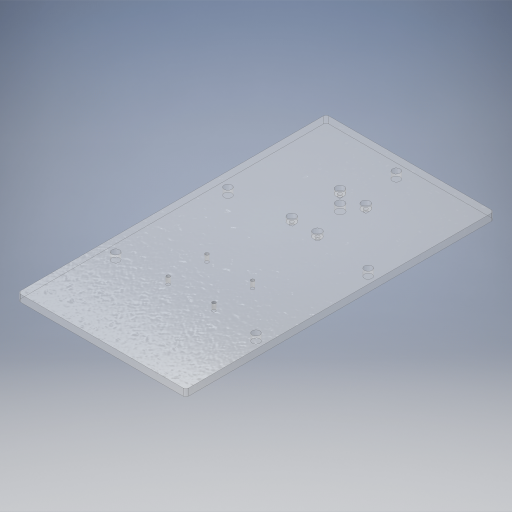
# Autodesk Inventor part: BT002_trajan20_21
Saved by Autodesk Inventor 2023 (Build 270158000, 158)
## iProperties
Company: HTBLA Kaindorf
RuleStatus: InUse
Created: 2022-08-03
Part Number: BT002_trajan20_21
Project: Zeichenmaschine_v2
Material: Acryl
Description: Platte Getriebemotor
Document SubType Name: Modeling
Designer: trajan20
Density: 1.188 g/cm^3
Appearance: Transparent - farblos
Mass: 155.33 g
Surface Area: 567.811 cm^2
Volume: 130.749 cm^3
AfterDocNew0: iProperties-Editor_aufrufen
Author: jan
Keywords: 2021
Autodesk Inventor part; units mm, degrees
ref_plane "YZ Plane" through (0, 0, 0) normal (1, 0, 0) x (0, 1, 0)
ref_plane "XZ Plane" through (0, 0, 0) normal (0, 1, 0) x (-1, 0, 0)
ref_plane "XY Plane" through (0, 0, 0) normal (0, 0, 1) x (1, 0, 0)
derived "BT000_trajan20_22_Zeichenmaschine_neu_Masterskizze.ipt"
sketch "Skizze3" plane through (0, 0, 0) normal (0, 0, 1) x (1, 0, 0)
  line L0 (0, 0) -> (-110, 0)
  line L1 (-220, 0) -> (-220, 120)
  line L2 (-220, 120) -> (0, 120)
  line L3 (0, 120) -> (0, 0)
  line L4 (-248.2253, 60) -> (-229.9902, 60) construction
  line L5 (-179.05, 50.815) -> (-179.05, 69.185) construction
  line L6 (-179.05, 69.185) -> (-144.68, 69.185) construction
  line L7 (-144.68, 50.3276) -> (-144.68, 69.185) construction
  line L8 (-143.2541, 50.815) -> (-179.05, 50.815) construction
  circle A0 centre (-170, 60) radius 3
  line L9 (-95, 40) -> (-70, 40)
  line L10 (-70, 40) -> (-70, 80)
  line L11 (-70, 80) -> (-95, 80)
  line L12 (-95, 80) -> (-95, 40)
  line L13 (-110, -37.5982) -> (-110, -22.8575) construction
  line L14 (-110, 0) -> (-220, 0)
  circle A1 centre (-170, 60) radius 20.5
  point P0 (-220, 60)
  point P1 (-144.68, 50.815)
  point P2 (-95, 60)
  point P3 (-91.3, 43.7)
  point P4 (-210, 60)
  point P5 (-110, 120)
  point P6 (-165, 0)
  point P7 (-60, 10)
  point P8 (-140, 10)
  point P9 (-140, 110)
  point P10 (-60, 110)
  point P11 (-60, 10)
  dimension "d4" = 120
  dimension "d5" = 220
  dimension "d6" = 50
  dimension "d8" = 9.05
  dimension "d9" = 34.37
  dimension "d11" = 9.185
  dimension "d12" = 18.37
  dimension "d17" = 6
  dimension "d18" = 40
  dimension "d19" = 25
  dimension "d20" = 75
  dimension "d21" = 3.7
  dimension "d22" = 3.7
  dimension "d39" = 10
  dimension "d40" = 10
  dimension "d41" = 10
  dimension "d42" = 10
  dimension "d43" = 10
  dimension "d51" = 80
  dimension "d52" = 80
  dimension "d53" = 41
  dimension "d64" = 60
  constraints: 34 end point, 10 point on line, 6 horizontal, 5 parallel, 4 midpoint, 3 coincident, 3 perpendicular, 3 vertical, 2 centre point, 1 vertical alignment
  measures "d4" distance between parallel lines of L0 L2
  measures "d5" distance between parallel lines of L1 L3
  measures "d6" distance from line of L1 point (-170, 60)
  measures "d8" distance from line of L5 point (-170, 60)
  measures "d9" distance between parallel lines of L5 L7
  measures "d11" distance from line of L6 point (-170, 60)
  measures "d12" distance between parallel lines of L8 L6
  measures "d17" diameter of A0
  measures "d18" distance between parallel lines of L11 L9
  measures "d19" distance between parallel lines of L12 L10
  measures "d20" distance from line of point (-170, 60) L12
  measures "d21" distance from line of L12 point (-91.3, 43.7)
  measures "d22" distance from line of L9 point (-91.3, 43.7)
  measures "d39" distance from line of L1 point (-210, 60)
  measures "d40" distance from line of L2 point (-60, 110)
  measures "d41" distance from line of L0 point (-60, 10)
  measures "d42" distance from line of L14 point (-140, 10)
  measures "d43" distance from line of L2 point (-140, 110)
  measures "d51" distance from line of L1 point (-140, 10)
  measures "d52" distance from line of L1 point (-140, 110)
  measures "d53" diameter of A1
  measures "d64" distance from line of L3 point (-60, 10)
extrude "Extrusion3" add sketch "Skizze3" against normal blind 5 contours L0 L14 L1 L2 L3 | L12 L11 L10 L9 | A1
hole "Bohrung1" at (-91.3, 43.7, 0) direction (0, 0, -1) diameter 2.459 end through all thread size "M3x0.5" class "6H" standard "ISO Metric profile"
pattern_linear "Rechteckige Anordnung1" count 2 spacing 32.6 along (0, 1, 0) count 2 spacing 27.6 along (1, 0, 0) of "Bohrung1"
fillet "Rundung1" radius 2 4 edges at (-220, 120, -2.5) (-220, 0, -2.5) (0, 120, -2.5) (0, 0, -2.5)
hole "Bohrung2" at (-210, 60, 0) at (-60, 10, 0) at (-140, 10, 0) at (-140, 110, 0) at (-60, 110, 0) direction (0, 0, -1) diameter 5.5 end through all
hole "Bohrung3" at (-179.05, 69.185, 0) at (-179.05, 50.815, 0) at (-144.68, 50.815, 0) at (-144.68, 69.185, 0) direction (0, 0, -1) diameter 2.7 end through all counterbore diameter 6 counterbore depth 3.2
equation "\"d4\" = Basis_Zubau_Breite_Profillänge + 4 * AluProfil_Abstand"
equation "\"d5\" = Basis_Zubau_Länge_Profillänge + 2 * AluProfil_Abstand"
equation "\"d22\" = d21"
equation "\"d41\" = d40"
equation "\"d42\" = d41"
equation "\"d43\" = d42"
equation "\"d34\" = d18 - 2 * d22"
equation "\"Basis_Zubau_Breite_Profillänge\" = 80"
equation "\"AluProfil_Abstand\" = 10"
equation "\"Basis_Zubau_Länge_Profillänge\" = 200"
